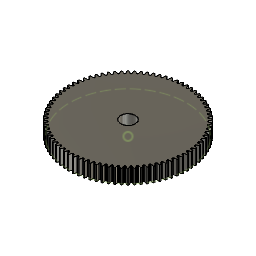
gear_mare (Autodesk Fusion 360 design; units mm, degrees)
part number: 2026-06-01-18-08-30-536
Autodesk Fusion 360 part; units mm, degrees
sketch "Base Circle" plane through (0, 0, 0) normal (0, 0, 1) x (1, 0, 0)
  circle A0 centre (0, 0) radius 38.843
  circle A1 centre (0, 0) radius 5
extrude "Extrude1" add sketch "Base Circle" along normal blind 10
sketch "Gear Tooth" plane through (0, 0, 0) normal (0, 0, 1) x (1, 0, 0)
  spline S0 degree 5 poles (37.5661, -1.2745) (37.576, -1.2745) (37.5958, -1.2743) (37.6254, -1.2737) (37.665, -1.2726) (37.7145, -1.2705) (37.764, -1.2677) (37.8134, -1.2641) (37.8629, -1.26) (37.9124, -1.2552) (37.9618, -1.2498) (38.0113, -1.244) (38.0608, -1.2377) (38.1102, -1.2311) (38.1597, -1.2241) (38.2091, -1.2167) (38.2585, -1.209) (38.3079, -1.201) (38.3573, -1.1926) (38.4067, -1.1838) (38.4561, -1.1748) (38.5054, -1.1654) (38.5548, -1.1557) (38.6041, -1.1457) (38.6534, -1.1355) (38.7027, -1.1249) (38.752, -1.1141) (38.8013, -1.103) (38.8506, -1.0917) (38.8998, -1.0801) (38.949, -1.0682) (38.9983, -1.0561) (39.0474, -1.0437) (39.0966, -1.0311) (39.1458, -1.0182) (39.1949, -1.0051) (39.2441, -0.9918) (39.2932, -0.9782) (39.3422, -0.9644) (39.3913, -0.9504) (39.4404, -0.9361) (39.4894, -0.9217) (39.5384, -0.907) (39.5874, -0.8921) (39.6364, -0.8769) (39.6853, -0.8616) (39.7342, -0.8461) (39.7831, -0.8303) (39.832, -0.8143) (39.8809, -0.7982) (39.9297, -0.7818) (39.9786, -0.7653) (40.0274, -0.7485) (40.0761, -0.7315) (40.1249, -0.7144) (40.1736, -0.697) (40.2223, -0.6795) (40.271, -0.6618) (40.3197, -0.6439) (40.3683, -0.6258) (40.4169, -0.6075) (40.4655, -0.589) (40.5141, -0.5703) (40.5626, -0.5515) (40.6111, -0.5325) (40.6596, -0.5133) (40.7081, -0.4939) (40.7565, -0.4743) (40.8049, -0.4546) (40.8533, -0.4347) (40.9017, -0.4146) (40.9403, -0.3984) (40.9693, -0.3861) (40.9886, -0.3779) (40.9983, -0.3738) knots 0 0 0 0 0 0 0.01428571 0.02857143 0.04285714 0.05714286 0.07142857 0.08571429 0.1 0.11428571 0.12857143 0.14285714 0.15714286 0.17142857 0.18571429 0.2 0.21428571 0.22857143 0.24285714 0.25714286 0.27142857 0.28571429 0.3 0.31428571 0.32857143 0.34285714 0.35714286 0.37142857 0.38571429 0.4 0.41428571 0.42857143 0.44285714 0.45714286 0.47142857 0.48571429 0.5 0.51428571 0.52857143 0.54285714 0.55714286 0.57142857 0.58571429 0.6 0.61428571 0.62857143 0.64285714 0.65714286 0.67142857 0.68571429 0.7 0.71428571 0.72857143 0.74285714 0.75714286 0.77142857 0.78571429 0.8 0.81428571 0.82857143 0.84285714 0.85714286 0.87142857 0.88571429 0.9 0.91428571 0.92857143 0.94285714 0.95714286 0.97142857 0.98571429 1 1 1 1 1 1
  spline S1 degree 5 poles (37.5661, 1.2745) (37.576, 1.2745) (37.5958, 1.2743) (37.6254, 1.2737) (37.665, 1.2726) (37.7145, 1.2705) (37.764, 1.2677) (37.8134, 1.2641) (37.8629, 1.26) (37.9124, 1.2552) (37.9618, 1.2498) (38.0113, 1.244) (38.0608, 1.2377) (38.1102, 1.2311) (38.1597, 1.2241) (38.2091, 1.2167) (38.2585, 1.209) (38.3079, 1.201) (38.3573, 1.1926) (38.4067, 1.1838) (38.4561, 1.1748) (38.5054, 1.1654) (38.5548, 1.1557) (38.6041, 1.1457) (38.6534, 1.1355) (38.7027, 1.1249) (38.752, 1.1141) (38.8013, 1.103) (38.8506, 1.0917) (38.8998, 1.0801) (38.949, 1.0682) (38.9983, 1.0561) (39.0474, 1.0437) (39.0966, 1.0311) (39.1458, 1.0182) (39.1949, 1.0051) (39.2441, 0.9918) (39.2932, 0.9782) (39.3422, 0.9644) (39.3913, 0.9504) (39.4404, 0.9361) (39.4894, 0.9217) (39.5384, 0.907) (39.5874, 0.8921) (39.6364, 0.8769) (39.6853, 0.8616) (39.7342, 0.8461) (39.7831, 0.8303) (39.832, 0.8143) (39.8809, 0.7982) (39.9297, 0.7818) (39.9786, 0.7653) (40.0274, 0.7485) (40.0761, 0.7315) (40.1249, 0.7144) (40.1736, 0.697) (40.2223, 0.6795) (40.271, 0.6618) (40.3197, 0.6439) (40.3683, 0.6258) (40.4169, 0.6075) (40.4655, 0.589) (40.5141, 0.5703) (40.5626, 0.5515) (40.6111, 0.5325) (40.6596, 0.5133) (40.7081, 0.4939) (40.7565, 0.4743) (40.8049, 0.4546) (40.8533, 0.4347) (40.9017, 0.4146) (40.9403, 0.3984) (40.9693, 0.3861) (40.9886, 0.3779) (40.9983, 0.3738) knots 0 0 0 0 0 0 0.01428571 0.02857143 0.04285714 0.05714286 0.07142857 0.08571429 0.1 0.11428571 0.12857143 0.14285714 0.15714286 0.17142857 0.18571429 0.2 0.21428571 0.22857143 0.24285714 0.25714286 0.27142857 0.28571429 0.3 0.31428571 0.32857143 0.34285714 0.35714286 0.37142857 0.38571429 0.4 0.41428571 0.42857143 0.44285714 0.45714286 0.47142857 0.48571429 0.5 0.51428571 0.52857143 0.54285714 0.55714286 0.57142857 0.58571429 0.6 0.61428571 0.62857143 0.64285714 0.65714286 0.67142857 0.68571429 0.7 0.71428571 0.72857143 0.74285714 0.75714286 0.77142857 0.78571429 0.8 0.81428571 0.82857143 0.84285714 0.85714286 0.87142857 0.88571429 0.9 0.91428571 0.92857143 0.94285714 0.95714286 0.97142857 0.98571429 1 1 1 1 1 1
  arc A0 (40.9983, -0.3738) -> (40.9983, 0.3738) centre (0, 0) ccw
  line L0 (37.5661, 1.2745) -> (37.5661, -1.2745)
  point P0 (37.8103, -1.2642)
  point P1 (38.055, -1.2384)
  point P2 (38.3, -1.2022)
  point P3 (38.5453, -1.1575)
  point P4 (38.7906, -1.1054)
  point P5 (39.0361, -1.0465)
  point P6 (39.2816, -0.9814)
  point P7 (39.5271, -0.9103)
  point P8 (39.7726, -0.8337)
  point P9 (40.018, -0.7517)
  point P10 (40.2633, -0.6645)
  point P11 (40.5085, -0.5724)
  point P12 (40.7535, -0.4755)
  point P13 (37.8103, 1.2642)
  point P14 (38.055, 1.2384)
  point P15 (38.3, 1.2022)
  point P16 (38.5453, 1.1575)
  point P17 (38.7906, 1.1054)
  point P18 (39.0361, 1.0465)
  point P19 (39.2816, 0.9814)
  point P20 (39.5271, 0.9103)
  point P21 (39.7726, 0.8337)
  point P22 (40.018, 0.7517)
  point P23 (40.2633, 0.6645)
  point P24 (40.5085, 0.5724)
  point P25 (40.7535, 0.4755)
extrude "Extrude2" add sketch "Gear Tooth" along normal blind 10
fillet "Fillet1" radius 0.5 2 edges at (38.8275, 1.097, 5) (38.8275, -1.097, 5)
pattern_circular "C-Pattern1" count 80 over 360 about axis through (0, 0, 0) along (0, 0, 1) of "Extrude2", "Fillet1"
sketch "Diametrial Pitch Circle" plane through (0, 0, 0) normal (0, 0, 1) x (1, 0, 0)
  circle A0 centre (0, 0) radius 40 construction
named bodies: "Spur Gear (80 teeth)"
